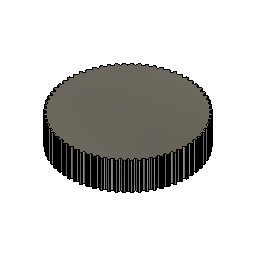
gear_68z (Autodesk Fusion 360 design; units mm, degrees)
Autodesk Fusion 360 part; units mm, degrees
sketch "Sketch1" plane through (0, 0, 0) normal (0, 0, 1) x (1, 0, 0) in component "gt2 pulley"
  circle A0 centre (0, 0) radius 21.6451 construction
  circle A1 centre (0, 0) radius 20.6411 construction
  line L0 (0, 0) -> (0, 21.6451) construction
  line L1 (0, 0) -> (0.9996, 21.622) construction
  line L2 (0, 0) -> (1.4056, 21.5994) construction
  circle A2 centre (0, 0) radius 21.3911 construction
  arc A3 (0.3934, 21.2535) -> (0.4673, 20.9584) centre (1.3891, 21.3459) ccw
  circle A4 centre (0, 0) radius 21.2411 construction
  arc A5 (0.2457, 21.3897) -> (0, 21.3911) centre (0, 0) ccw
  arc A6 (0.3934, 21.2535) -> (0.2457, 21.3897) centre (0.244, 21.2397) ccw
  arc A7 (0.4673, 20.9584) -> (0.9533, 20.619) centre (0.9789, 21.1735) ccw
  arc A8 (0, 21.3911) -> (-0.2457, 21.3897) centre (0, 0) ccw
  arc A9 (-0.2457, 21.3897) -> (-0.3934, 21.2535) centre (-0.244, 21.2397) ccw
  arc A10 (-0.4673, 20.9584) -> (-0.3934, 21.2535) centre (-1.3891, 21.3459) ccw
  arc A11 (-0.9533, 20.619) -> (-0.4673, 20.9584) centre (-0.9789, 21.1734) ccw
  arc A12 (0.9533, 20.619) -> (-0.9533, 20.619) centre (0, 0) ccw
  point P0 (1.3891, 21.3459)
  point P1 (0, 21.3911)
  dimension "d18" = 43.2901
  dimension "d19" = 2.647
  dimension "d22" = 1.004
  dimension "d24" = 0.75
  dimension "d26" = 1
  dimension "d27" = 0.15
  dimension "d28" = 0.15
  dimension "d47" = 0.555
  dimension "d52" = 3.812
  constraint coincident A0.centre A1.centre
  constraint coincident A0 L0.end
  constraint vertical L0
  constraint coincident A0 L1.end
  constraint coincident A0 L2.end
  constraint concentric A1 A2
  constraint coincident A1 A7.end
  constraint coincident L1 A7.end
  constraint coincident A2 P0
  constraint coincident L2 P0
  constraint coincident P0 A3.centre
  constraint coincident A2 P1
  constraint coincident L0 P1
  constraint concentric A2 A4
  constraint coincident P1 A5.end
  constraint coincident A4 A6.centre
  constraint coincident A3.start A6.start
  constraint tangent A3 A6
  constraint tangent A3 A7
  constraint symmetric L0 A7.end A11.start
  constraint symmetric L0 A3.start A9.end
  constraint symmetric L0 A3.end A10.start
  constraint symmetric L0 A3 A10
  constraint symmetric L0 A5.start A8.end
  constraint symmetric L0 P1 A5.end
  constraint symmetric L0 A5 A8
  constraint symmetric L0 A6 A9
  constraint symmetric L0 A7 A11
  constraint coincident A1 A11.start
  constraint tangent A1 A7
  constraint coincident L1 A7.centre
  measures "d18" diameter of A0
  measures "d19" angle of L0 L1
  measures "d22" distance of A0 A1
  measures "d24" distance of A1 A2
  measures "d26" radius of A3
  measures "d27" distance of A2 A4
  measures "d28" radius of A6
  measures "d47" radius of A7
extrude "Extrude1" add sketch "Sketch1" along normal blind 10 makes body 1
pattern_circular "C-Pattern1" count 68 over 360 about axis through (0, 0, 1.75) along (0, 0, 1) of bodies 1 makes body 2 at (-2.01, 20.543, 6.6667) makes body 3 at (-3.0614, 20.4128, 3.3333) makes body 4 at (-6.3583, 19.6374, 6.6667) makes body 5 at (-7.3575, 19.2852, 6.6667) makes body 6 at (-8.5308, 18.7957, 3.3333) makes body 7 at (-10.9561, 17.4934, 6.6667) makes body 8 at (-13.0228, 16.0144, 6.6667) makes body 9 at (-14.4448, 14.7445, 6.6667) makes body 10 at (-14.7445, 14.4448, 3.3333) makes body 11 at (-16.5356, 12.3543, 6.6667) makes body 12 at (-17.1477, 11.4896, 3.3333) makes body 13 at (-18.1347, 9.8584, 3.3333) makes body 14 at (-18.9669, 8.1431, 3.3333) makes body 15 at (-19.8239, 5.7505, 6.6667) makes body 16 at (-20.3088, 3.6886, 6.6667) makes body 17 at (-20.6082, 1.1649, 6.6667) makes body 18 at (-20.6277, 0.7415, 3.3333) makes body 19 at (-20.543, -2.01, 6.6667) makes body 20 at (-20.2699, -3.8969, 6.6667) makes body 21 at (-19.6374, -6.3583, 6.6667) makes body 22 at (-19.2087, -7.5551, 6.6667) makes body 23 at (-18.7957, -8.5308, 3.3333) makes body 24 at (-17.4934, -10.9561, 6.6667) makes body 25 at (-16.0144, -13.0228, 6.6667) makes body 26 at (-15.1823, -13.9839, 6.6667) makes body 27 at (-13.8273, -15.3251, 6.6667) makes body 28 at (-13.0228, -16.0144, 3.3333) makes body 29 at (-10.2286, -17.9284, 6.6667) makes body 30 at (-9.8584, -18.1347, 3.3333) makes body 31 at (-8.1431, -18.9669, 6.6667) makes body 32 at (-5.7505, -19.8239, 6.6667) makes body 33 at (-3.6886, -20.3088, 6.6667) makes body 34 at (-2.6417, -20.4713, 3.3333) makes body 35 at (-0.7415, -20.6277, 3.3333) makes body 36 at (2.01, -20.543, 6.6667) makes body 37 at (3.8969, -20.2699, 6.6667) makes body 38 at (4.9318, -20.0432, 3.3333) makes body 39 at (6.7601, -19.5027, 6.6667) makes body 40 at (8.5308, -18.7957, 3.3333) makes body 41 at (11.4896, -17.1477, 6.6667) makes body 42 at (12.5234, -16.4079, 6.6667) makes body 43 at (14.4448, -14.7445, 6.6667) makes body 44 at (14.7445, -14.4448, 3.3333) makes body 45 at (16.5356, -12.3543, 6.6667) makes body 46 at (17.1477, -11.4896, 3.3333) makes body 47 at (18.1347, -9.8584, 3.3333) makes body 48 at (18.9669, -8.1431, 3.3333) makes body 49 at (19.8239, -5.7505, 6.6667) makes body 50 at (20.3088, -3.6886, 6.6667) makes body 51 at (20.6082, -1.1649, 6.6667) makes body 52 at (20.6277, -0.7415, 3.3333) makes body 53 at (20.543, 2.01, 6.6667) makes body 54 at (20.4128, 3.0614, 3.3333) makes body 55 at (19.6374, 6.3583, 6.6667) makes body 56 at (19.5027, 6.7601, 6.6667) makes body 57 at (18.7957, 8.5308, 3.3333) makes body 58 at (17.4934, 10.9561, 6.6667) makes body 59 at (16.0144, 13.0228, 6.6667) makes body 60 at (15.1823, 13.9839, 6.6667) makes body 61 at (14.4448, 14.7445, 3.3333) makes body 62 at (12.3543, 16.5356, 6.6667) makes body 63 at (11.4896, 17.1477, 3.3333) makes body 64 at (9.1055, 18.5241, 6.6667) makes body 65 at (7.5551, 19.2087, 6.6667) makes body 66 at (5.7505, 19.8239, 6.6667) makes body 67 at (4.5193, 20.1403, 3.3333) makes body 68 at (2.6417, 20.4713, 3.3333)
sketch "Sketch2" plane through (0, 0, 10) normal (0, 0, 1) x (-1, 0, 0)
  arc A0 (-18.2772, -10.8541) -> (-18.3152, -11.0513) centre (-18.1868, -10.9738) ccw
  arc A1 (-18.3152, -11.0513) -> (-18.0565, -11.4691) centre (0, 0) ccw
  arc A2 (-18.0565, -11.4691) -> (-17.863, -11.523) centre (-17.9299, -11.3887) ccw
  arc A3 (-17.5732, -11.4304) -> (-17.863, -11.523) centre (-17.4174, -12.4182) ccw
  arc A4 (-17.0288, -11.665) -> (-17.5732, -11.4305) centre (-17.4867, -11.9787) ccw
  arc A5 (-18.0325, -10.044) -> (-17.0288, -11.665) centre (0, 0) ccw
  arc A6 (-18.0651, -10.6359) -> (-18.0325, -10.044) centre (-18.5174, -10.3141) ccw
  arc A7 (-18.2772, -10.8541) -> (-18.0651, -10.6359) centre (-18.8799, -10.0561) ccw
  circle A8 centre (0, 0) radius 20.6411
  constraint concentric A1 A8
extrude "Extrude2" add sketch "Sketch2" against normal blind 10 contours A5 A8 bodies 1 2 3 4 5 6 7 8 9 10 11 12 13 14 15 16 17 18 19 20 21 22 23 24 25 26 27 28 29 30 31 32 33 34 35 36 37 38 39 40 41 42 43 44 45 46 47 48 49 50 51 52 53 54 55 56 57 58 59 60 61 62 63 64 65 66 67 68
extrude "Extrude4" [suppressed] in component "gt2 pulley"
pattern_circular "C-Pattern7" [suppressed] in component "gt2 pulley"
extrude "Extrude3" [suppressed] in component "gt2 pulley"
pattern_circular "C-Pattern6" [suppressed] in component "gt2 pulley"
extrude "Extrude2'" [suppressed] in component "gt2 pulley"
pattern_circular "C-Pattern5" [suppressed] in component "gt2 pulley"
extrude "Extrude1'" [suppressed] in component "gt2 pulley"
pattern_circular "C-Pattern4" [suppressed] in component "gt2 pulley"
pattern_circular "C-Pattern3" [suppressed] in component "gt2 pulley"
pattern_circular "C-Pattern2" [suppressed] in component "gt2 pulley"
pattern_circular "C-Pattern1'" [suppressed] in component "gt2 pulley"
copy_body "Body->Comp1" [suppressed] in component "Component"
copy_body "Body->Comp2" [suppressed] in component "Component'"
copy_body "Body->Comp3" [suppressed] in component "Component''"
copy_body "Body->Comp4" [suppressed] in component "Component'''"
copy_body "Body->Comp5" [suppressed] in component "Component''''"
copy_body "Body->Comp6" [suppressed] in component "Component'''''"
copy_body "Body->Comp7" [suppressed] in component "Component''''''"
copy_body "Body->Comp8" [suppressed] in component "Component'''''''"
copy_body "Body->Comp9" [suppressed] in component "Component''''''''"
copy_body "Body->Comp10" [suppressed] in component "Component'''''''''"
copy_body "Body->Comp11" [suppressed] in component "Component''''''''''"
copy_body "Body->Comp12" [suppressed] in component "Component'''''''''''"
copy_body "Body->Comp13" [suppressed] in component "Component''''''''''''"
copy_body "Body->Comp14" [suppressed] in component "Component'''''''''''''"
copy_body "Body->Comp15" [suppressed] in component "Component''''''''''''''"
copy_body "Body->Comp16" [suppressed] in component "Component'''''''''''''''"
copy_body "Body->Comp17" [suppressed] in component "Component''''''''''''''''"
copy_body "Body->Comp18" [suppressed] in component "Component'''''''''''''''''"
copy_body "Body->Comp19" [suppressed] in component "Component''''''''''''''''''"
copy_body "Body->Comp20" [suppressed] in component "Component'''''''''''''''''''"
component "gt2 pulley" placed x (1, 0, 0) y (0, 1, 0) z (0, 0, 1) at (0, 0, 0)
equation "NumTeeth = 68" comment "min 20"
equation "ToothPitch = 2 mm"
equation "PullyDia = NumTeeth * ToothPitch / PI"
equation "ToothAng = ( ( 360 / NumTeeth ) * 1 deg )"
equation "TransOffsetAngle = ToothAng * 0.2"
equation "Sholulder_Radius = 0.15 mm"
equation "Root_Radius = 0.555 mm"
equation "TransRadius = 1 mm"
equation "ToolHeight = 0.75 mm"
equation "PLD = 0.254 mm"
equation "d18 = PullyDia"
equation "d19 = ToothAng / 2"
equation "d22 = PLD + ToolHeight"
equation "d24 = ToolHeight"
equation "d26 = TransRadius"
equation "d27 = Sholulder_Radius"
equation "d31 = NumTeeth"
equation "d33 = NumTeeth"
equation "d35 = NumTeeth"
equation "d37 = NumTeeth"
equation "d41 = NumTeeth"
equation "d45 = NumTeeth"
equation "d47 = Root_Radius"
equation "d50 = NumTeeth"
